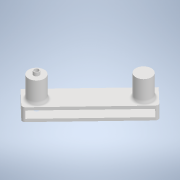
# Autodesk Inventor part: Base
Saved by Autodesk Inventor 2022 (Build 260153000, 153)
## iProperties
Created: 2022-05-19
Part Number: Base
Material: Generic
Document SubType Name: Modeling
Designer: abdoo
Density: 1 g/cm^3
Appearance: Default
Author: abdoo
Autodesk Inventor part; units mm, degrees
ref_plane "YZ Plane" through (0, 0, 0) normal (1, 0, 0) x (0, 1, 0)
ref_plane "XZ Plane" through (0, 0, 0) normal (0, 1, 0) x (-1, 0, 0)
ref_plane "XY Plane" through (0, 0, 0) normal (0, 0, 1) x (1, 0, 0)
sketch "Sketch1" plane through (0, 0, 0) normal (0, 1, 0) x (-1, 0, 0)
  line L0 (0, 0) -> (100, 0)
  line L1 (100, 0) -> (100, -50)
  line L2 (100, -50) -> (0, -50)
  line L3 (0, -50) -> (0, 0)
  dimension "d0" = 100
  dimension "d1" = 50
  constraints: 8 end point, 2 parallel, 1 horizontal, 1 perpendicular
  measures "d0" distance of L1.end L2.end
  measures "d1" distance of L0.end L1.end
extrude "Extrusion1" add sketch "Sketch1" along normal blind 3
sketch "Sketch2" plane through (0, 3, 0) normal (0, 1, 0) x (1, 0, 0)
  circle A0 centre (-82.0522, 25) radius 7
  circle A1 centre (-27.5493, 25) radius 7
  line L0 (-100, 50) -> (-100, 0) projected
  line L1 (0, 0) -> (0, 50) projected
  line L2 (0, 50) -> (-100, 50) projected
  dimension "d4" = 14
  dimension "d5" = 14
  dimension "d6" = 17.9478
  dimension "d7" = 27.5493
  dimension "d8" = 25
  dimension "d9" = 25
  constraints: 2 centre point
  measures "d4" diameter of A0
  measures "d5" diameter of A1
  measures "d6" distance from line of A0.centre L0
  measures "d7" distance from line of A1.centre L1
  measures "d8" distance from line of L2 A1.centre
  measures "d9" distance from line of A0.centre L2
extrude "Extrusion2" add sketch "Sketch2" along normal blind 18
sketch "Sketch3" plane through (-82.0522, 21, -25) normal (0, 1, 0) x (1, 0, 0)
  circle A0 centre (0, 0) radius 7 projected
  circle A1 centre (54.5029, 0) radius 7 projected
  circle A2 centre (0, 0) radius 2.875
  circle A3 centre (54.5029, 0) radius 2.45
  point P0 (82.0522, -25)
  dimension "d12" = 5.75
  dimension "d13" = 4.9
  constraints: 2 centre point, 2 coincident
  measures "d12" diameter of A2
  measures "d13" diameter of A3
extrude "Extrusion3" add sketch "Sketch3" along normal blind 3 contours A2 | A3
sketch "Sketch5" plane through (-27.5493, 24, -25) normal (0, 1, 0) x (1, 0, 0)
  circle A0 centre (0, 0) radius 1.925
  point P0 (27.5493, -25)
  dimension "d20" = 3.85
  constraints: 1 centre point
  measures "d20" diameter of A0
extrude "Extrusion5" cut sketch "Sketch5" against normal up to surface (24 mm away)
sketch "Sketch7" plane through (0, 0, 0) normal (0, -1, 0) x (1, 0, 0)
  line L0 (2.4404, 5.5552) -> (-105.2601, 5.5552)
  line L1 (-105.2601, 5.5552) -> (-105.2601, -59.9514)
  line L2 (-105.2601, -59.9514) -> (2.4404, -59.9514)
  line L3 (2.4404, -59.9514) -> (2.4404, 5.5552)
  circle A0 centre (-27.5493, -25) radius 2.45 projected
  circle A1 centre (-27.5493, -25) radius 7 projected
  point P0 (0, 0)
  constraints: 8 end point, 2 parallel, 1 horizontal, 1 perpendicular
extrude "Extrusion6" cut sketch "Sketch7" against normal blind 50 contours L3 L2 L1 L0
ref_plane "Work Plane1" through (-108.1719, 0, -146.2869) normal (0, 1, 0) x (0.6910823, 0, -0.7227761)
sketch "Sketch8" plane through (-108.1719, 0, -146.2869) normal (0, 1, 0) x (0.6910823, 0, -0.7227761)
  line L0 (-40.64, -147.32) -> (40.64, -147.32) projected
  line L1 (-40.64, 147.32) -> (-40.64, -147.32) projected
  line L2 (-43.34, -130.02) -> (-40.84, -130.02)
  line L3 (-40.84, -130.02) -> (-40.84, -150.02)
  line L4 (-40.84, -150.02) -> (-43.34, -150.02)
  line L5 (-43.34, -150.02) -> (-43.34, -130.02)
  line L6 (-23.34, -147.52) -> (-40.84, -147.52)
  line L7 (-40.84, -147.52) -> (-40.84, -150.02)
  line L8 (-23.34, -147.52) -> (-23.34, -150.02)
  line L9 (-23.34, -150.02) -> (-40.84, -150.02)
  line L10 (-40.84, -130.02) -> (-23.34, -130.02)
  line L11 (-23.34, -130.02) -> (-23.34, -147.52)
  arc A0 (-33.6873, -142.3194) -> (-35.0746, -141.7135) centre (-33.64, -140.32) ccw projected
  circle A1 centre (-33.64, -140.32) radius 3.8 projected
  circle A2 centre (-31.9463, -142.0913) radius 7 projected
  point P0 (-30.9769, -179.2803)
  point P1 (-40.84, -150.02)
  dimension "d26" = 0.2
  dimension "d27" = 0.2
  dimension "d29" = 20
  dimension "d30" = 2.5
  dimension "d31" = 2.5
  dimension "d32" = 20
  constraints: 20 end point, 4 perpendicular, 2 horizontal, 2 parallel, 1 point on line
  measures "d26" distance between parallel lines of L3 L1
  measures "d27" distance between parallel lines of L6 L0
  measures "d29" distance of L4.end L2.start
  measures "d30" distance between parallel lines of L5 L3
  measures "d31" distance of L6.start L8.end
  measures "d32" distance between parallel lines of L5 L8
extrude "Extrusion7" add sketch "Sketch8" along normal blind 2.5 contours L1 L10 L11 L0 A2 | L0 A2 L6 L3 L10 L1 | L0 L11 L6 A2 | A2 L6 L8 L9 L3 | L3 L4 L5 L2
sketch "Sketch9" plane through (0, 0, 0) normal (0, -1, 0) x (1, 0, 0)
  line L0 (-29.6926, -11.2856) -> (-15.8709, -25.7411) projected
  line L1 (-15.8709, -25.7411) -> (-17.6779, -27.4688)
  line L2 (-15.8709, -25.7411) -> (-30.3264, -39.5627) projected
  line L3 (-17.6779, -27.4688) -> (-31.4995, -13.0133)
  line L4 (-30.3264, -39.5627) -> (-44.1481, -25.1072) projected
  line L5 (-44.1481, -25.1072) -> (-42.4204, -26.9142)
  line L6 (-42.4204, -26.9142) -> (-29.7718, -14.8202)
  line L7 (-30.3264, -39.5627) -> (-44.1481, -25.1072) projected
  line L8 (-15.8709, -25.7411) -> (-30.3264, -39.5627) projected
  line L9 (-29.6926, -11.2856) -> (-15.8709, -25.7411) projected
  line L10 (-44.1481, -25.1072) -> (-29.6926, -11.2856) projected
  circle A0 centre (-27.5493, -25) radius 1.925 projected
  point P0 (0, 0)
  dimension "d35" = 2.5
  dimension "d36" = 0
  dimension "d37" = 2.5
  constraints: 8 end point, 2 point on line, 1 perpendicular
  measures "d35" distance of L0.end L1.end
  measures "d36" distance between parallel lines of L2 L1
  measures "d37" distance of L4.end L5.end
extrude "Extrusion8" add sketch "Sketch9" along normal blind 6.4 contours L0 L1 L3 L10 | L3 L6 L4 L10
sketch "Sketch10" plane through (0, -6.4, 0) normal (0, -1, 0) x (1, 0, 0)
  line L0 (-30.3264, -39.5627) -> (-44.1481, -25.1072) projected
  line L1 (-44.1481, -25.1072) -> (-29.6926, -11.2856) projected
  line L2 (-29.6926, -11.2856) -> (-15.8709, -25.7411) projected
  line L3 (-15.8709, -25.7411) -> (-30.3264, -39.5627) projected
  circle A0 centre (-27.5493, -25) radius 7 projected
  circle A1 centre (-27.5493, -25) radius 1.925 projected
  point P0 (0, 0)
extrude "Extrusion9" add sketch "Sketch10" along normal blind 2.5 contours L0 L1 L2 L3 | A0
fillet "Fillet1" radius 2.5 1 edges at (-29.6926, -3.2, -11.2856)
fillet "Fillet2" radius 2.5 1 edges at (-34.5493, 2.5, -25)
sketch "Sketch11" plane through (0, -8.9, 0) normal (0, -1, 0) x (1, 0, 0)
  circle A0 centre (-27.5493, -25) radius 1.925 projected
  arc A1 (-27.9649, -13.0925) -> (-31.4995, -13.0133) centre (-29.7718, -14.8202) ccw projected
  line L0 (-31.4995, -13.0133) -> (-44.1481, -25.1072) projected
  line L1 (-44.1481, -25.1072) -> (-30.3264, -39.5627) projected
  line L2 (-30.3264, -39.5627) -> (-15.8709, -25.7411) projected
  line L3 (-15.8709, -25.7411) -> (-27.9649, -13.0925) projected
  circle A2 centre (-27.5493, -25) radius 2.45 projected
  line L4 (-28.8768, -29.5443) -> (-32.1485, -26.1225)
  line L5 (-32.1485, -26.1225) -> (-30.821, -21.5782)
  line L6 (-30.821, -21.5782) -> (-26.2218, -20.4557)
  line L7 (-26.2218, -20.4557) -> (-22.95, -23.8775)
  line L8 (-22.95, -23.8775) -> (-24.2775, -28.4218)
  line L9 (-24.2775, -28.4218) -> (-28.8768, -29.5443)
  line L10 (-15.8709, -25.7411) -> (-27.9649, -13.0925) projected
  point P0 (0, 0)
  dimension "d44" = 8.2
  constraints: 12 end point, 1 coincident, 1 parallel, 13 other
  measures "d44" distance between parallel lines of L4 L7
extrude "Extrusion10" cut sketch "Sketch11" against normal blind 1.5 contours L4 L5 L6 L7 L8 L9
sketch "Sketch12" plane through (-30.3264, 0, -39.5627) normal (0.6910823, 0, -0.7227761) x (-0.7227761, 0, -0.6910823)
  line L0 (-17.5, 0) -> (0, 0) projected
  line L1 (0, 0) -> (0, 2.5) projected
  line L2 (-20, 2.5) -> (-16.0939, 2.5) projected
  line L3 (-20, -8.9) -> (-20, 2.5) projected
  line L4 (0, -8.9) -> (-20, -8.9) projected
  line L5 (0, -6.4) -> (0, -8.9) projected
  line L6 (0, -6.4) -> (-17.5, -6.4) projected
  line L7 (-17.5, 0) -> (-17.5, -6.4) projected
  line L8 (-8.0488, 2.5) -> (0, 2.5) projected
  spline S0 degree 7 poles (-8.0488, 2.5) (-8.2834, 2.5) (-8.5183, 2.5046) (-8.7535, 2.5129) (-8.9887, 2.5241) (-9.2242, 2.5372) (-9.4597, 2.5515) (-10.0356, 2.5875) (-10.3761, 2.6096) (-10.7171, 2.6304) (-11.0588, 2.6476) (-11.4009, 2.6595) (-11.7433, 2.6654) (-12.423, 2.665) (-12.7602, 2.6588) (-13.0971, 2.6469) (-13.4335, 2.6298) (-13.7694, 2.6094) (-14.1047, 2.5877) (-14.6765, 2.5519) (-14.9131, 2.5375) (-15.1496, 2.5243) (-15.386, 2.513) (-15.6222, 2.5046) (-15.8582, 2.5) (-16.0939, 2.5) knots 0 0 0 0 0 0 0 0 0.20547 0.20547 0.20547 0.20547 0.20547 0.20547 0.50178 0.50178 0.50178 0.50178 0.50178 0.50178 0.793593 0.793593 0.793593 0.793593 0.793593 0.793593 1 1 1 1 1 1 1 1 projected
  point P0 (-49.2603, 0)
  constraints: 1 horizontal alignment
ref_plane "Work Plane2" through (-186.5657, -6, -277.4707) normal (0.6910823, 0, -0.7227761) x (0, 1, 0)
extrude "Extrusion11" add sketch "Sketch12" along normal blind 64.18
sketch "Sketch13" plane through (14.0272, 0, -85.9505) normal (0.6910823, 0, -0.7227761) x (-0.7227761, 0, -0.6910823)
  line L0 (0, 2.5) -> (-17.5, 2.5) projected
  line L1 (-17.5, -8.9) -> (0, -8.9) projected
  line L2 (0, -8.9) -> (0, 2.5) projected
  line L3 (-20, -8.9) -> (-20, 2.5) projected
  line L4 (-17.5, -6.4) -> (-17.5, 0) projected
  line L5 (-17.5, 0) -> (0, 0) projected
  line L6 (0, 0) -> (0, 2.5) projected
  line L7 (-16.0939, 2.5) -> (-20, 2.5) projected
  line L8 (-20, 2.5) -> (-20, -8.9) projected
  line L9 (-20, -8.9) -> (0, -8.9) projected
  line L10 (0, -8.9) -> (0, -6.4) projected
  line L11 (0, -6.4) -> (-17.5, -6.4) projected
  line L12 (0, 2.5) -> (-8.0488, 2.5) projected
  point P0 (-49.2603, 0)
  point P1 (-20, 2.5)
  constraints: 1 horizontal alignment
extrude "Extrusion12" add sketch "Sketch13" along normal blind 2.5
fillet "Fillet3" radius 2.5 1 edges at (30.2104, -3.2, -73.9358)
ref_plane "Work Plane3" through (-14.1966, -8.9, -56.4323) normal (-0.6910823, 0, 0.7227761) x (0.7227761, 0, 0.6910823)
mirror "Mirror1" about plane through (-14.1966, -8.9, -56.4323) normal (-0.6910823, 0, 0.7227761)
sketch "Sketch14" plane through (16.6058, 24, -71.1801) normal (0, 1, 0) x (1, 0, 0)
  circle A0 centre (0, 0) radius 1.925 projected
  circle A1 centre (0, 0) radius 1.925 projected
  circle A2 centre (0, 0) radius 2.45 projected
  point P0 (-16.6058, -71.1801)
ref_plane "Work Plane4" through (-246.9785, 21, -281.7123) normal (0, -1, 0) x (0.7227761, 0, 0.6910823)
extrude "Extrusion13" cut sketch "Sketch14" against normal up to surface (3 mm away)
sketch "Sketch15" plane through (16.6058, 21, -71.1801) normal (0, 1, 0) x (1, 0, 0)
  circle A0 centre (0, 0) radius 7 projected
  point P0 (-16.6058, -71.1801)
ref_plane "Work Plane5" through (-242.7369, 0, -277.4707) normal (0, 1, 0) x (-0.6910823, 0, 0.7227761)
extrude "Extrusion14" add sketch "Sketch15" against normal up to surface (21 mm away)
extrude "Extrusion15" cut sketch "Sketch11" against normal blind 1.5 contours A0 | A2 | L4 L5 L6 L7 L8 L9
extrude "Extrusion16" cut sketch "Sketch5" against normal up to surface (32.9 mm away)
sketch "Sketch16" plane through (-44.1481, -8.9, -25.1072) normal (-0.7227761, 0, -0.6910823) x (-0.6910823, 0, 0.7227761)
  line L0 (-84.18, 8.9) -> (-2.5, 8.9) projected
  line L1 (-84.18, 2.5) -> (-84.18, 8.9) projected
  line L2 (-2.5, 2.5) -> (-84.18, 2.5) projected
  line L3 (-2.5, 8.9) -> (-2.5, 2.5) projected
  point P0 (-12.3631, 8.9)
extrude "Extrusion17" cut sketch "Sketch16" against normal blind 20
body "Solid1"
